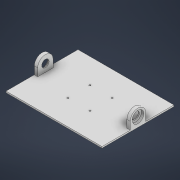
# Autodesk Inventor part: Testplatte_Differential
Saved by Autodesk Inventor 2021 (Build 250183000, 183)
## iProperties
Created: 2021-01-24
Part Number: Testplatte_Differential
Material: Generisch
Document SubType Name: Modeling
Designer: Ctroi
Density: 1 g/cm^3
Appearance: Vorgabe
Author: Ctroi
Autodesk Inventor part; units mm, degrees
ref_plane "YZ Plane" through (0, 0, 0) normal (1, 0, 0) x (0, 1, 0)
ref_plane "XZ Plane" through (0, 0, 0) normal (0, 1, 0) x (-1, 0, 0)
ref_plane "XY Plane" through (0, 0, 0) normal (0, 0, 1) x (1, 0, 0)
sketch "Skizze1" plane through (0, 0, 0) normal (0, 1, 0) x (-1, 0, 0)
  line L0 (100, -75) -> (-100, -75)
  line L1 (-100, -75) -> (-100, 75)
  line L2 (-100, 75) -> (100, 75)
  line L3 (100, 75) -> (100, -75)
  line L4 (0, -105) -> (0, 105) projected
  line L5 (-140, 0) -> (140, 0) projected
  point P0 (0, 0)
  dimension "d0" = 200
  dimension "d1" = 150
  constraints: 8 end point, 2 parallel, 1 horizontal, 1 perpendicular, 2 other
  measures "d0" distance of L1.end L2.end
  measures "d1" distance of L0.end L1.end
extrude "Extrusion1" add sketch "Skizze1" along normal blind 3
sketch "Skizze2" plane through (0, 3, 0) normal (0, 1, 0) x (1, 0, 0)
  line L0 (-93, 16) -> (-100, 16)
  line L1 (-100, 16) -> (-100, -16)
  line L2 (-100, -16) -> (-93, -16)
  line L3 (-93, -16) -> (-93, 16)
  line L4 (0, 105) -> (0, -105) projected
  line L5 (140, 0) -> (-140, 0) projected
  line L6 (-100, 75) -> (-100, -75) projected
  line L7 (93, 16) -> (100, 16)
  line L8 (100, 16) -> (100, -16)
  line L9 (100, -16) -> (93, -16)
  line L10 (93, -16) -> (93, 16)
  point P0 (0, 0)
  dimension "d4" = 7
  dimension "d5" = 32
  dimension "d6" = 0
  dimension "d58" = 32
  constraints: 16 end point, 4 symmetric about line, 2 parallel, 1 horizontal, 1 perpendicular, 1 other
  measures "d4" distance of L2.end L1.end
  measures "d5" distance of L1.end L0.end
  measures "d6" distance between parallel lines of L6 L1
  measures "d58" distance between parallel lines of L9 L7
extrude "Extrusion2" add sketch "Skizze2" along normal blind 32
sketch "Skizze3" plane through (-100, 0, -75) normal (-1, 0, 0) x (0, 0, 1)
  circle A0 centre (75, 19) radius 12.1
  line L0 (91, 3) -> (91, 35) projected
  line L1 (59, 35) -> (91, 35) projected
  point P0 (75, 0)
  dimension "d9" = 24.2
  dimension "d11" = 16
  dimension "d12" = 16
  constraints: 1 centre point
  measures "d9" diameter of A0
  measures "d11" distance from line of L0 A0.centre
  measures "d12" distance from line of L1 A0.centre
extrude "Extrusion4" cut sketch "Skizze3" against normal blind 5
sketch "Skizze4" plane through (100, 0, 75) normal (1, 0, 0) x (0, 0, -1)
  circle A0 centre (75, 19) radius 12.1
  line L0 (91, 3) -> (91, 35) projected
  line L1 (59, 35) -> (91, 35) projected
  point P0 (75, 0)
  dimension "d17" = 24.2
  dimension "d18" = 16
  dimension "d19" = 16
  constraints: 1 centre point
  measures "d17" diameter of A0
  measures "d18" distance from line of L0 A0.centre
  measures "d19" distance from line of L1 A0.centre
extrude "Extrusion5" cut sketch "Skizze4" against normal blind 5
sketch "Skizze5" plane through (95, 19, 0) normal (1, 0, 0) x (0, 0, -1)
  circle A0 centre (0, 0) radius 7.6
  line L0 (-16, 16) -> (16, 16) projected
  line L1 (-16, -16) -> (-16, 16) projected
  point P0 (0, -19)
  dimension "d22" = 15.2
  dimension "d23" = 16
  dimension "d24" = 16
  constraints: 1 centre point
  measures "d22" diameter of A0
  measures "d23" distance from line of L0 A0.centre
  measures "d24" distance from line of L1 A0.centre
sketch "Skizze6" plane through (-95, 19, 0) normal (-1, 0, 0) x (0, 0, 1)
  circle A0 centre (0, 0) radius 7.6
  line L0 (-16, 16) -> (16, 16) projected
  line L1 (16, -16) -> (16, 16) projected
  point P0 (0, -19)
  dimension "d25" = 15.2
  dimension "d26" = 16
  dimension "d27" = 16
  constraints: 1 centre point
  measures "d25" diameter of A0
  measures "d26" distance from line of L0 A0.centre
  measures "d27" distance from line of L1 A0.centre
extrude "Extrusion6" cut sketch "Skizze6" against normal up to surface (2 mm away)
extrude "Extrusion7" cut sketch "Skizze5" against normal up to surface (2 mm away)
sketch "Skizze11" plane through (0, 3, 0) normal (0, 1, 0) x (1, 0, 0)
  circle A0 centre (23, -23) radius 1.6
  circle A1 centre (23, 23) radius 1.6
  line L0 (140, 0) -> (-140, 0) projected
  line L1 (100, 16) -> (100, 75) projected
  line L2 (100, -75) -> (100, -16) projected
  line L3 (0, 105) -> (0, -105) projected
  circle A2 centre (-23, -23) radius 1.6
  circle A3 centre (-23, 23) radius 1.6
  circle A4 centre (23, 23) radius 1.6
  circle A5 centre (-23, 23) radius 1.6
  line L4 (100, 75) -> (-100, 75) projected
  point P0 (0, 0)
  dimension "d50" = 3.2
  dimension "d51" = 3.2
  dimension "d52" = 23
  dimension "d53" = 23
  dimension "d54" = 77
  dimension "d55" = 77
  dimension "d62" = 3.2
  dimension "d63" = 3.2
  dimension "d64" = 23
  dimension "d65" = 23
  dimension "d66" = 52
  dimension "d67" = 52
  constraints: 6 centre point, 2 symmetric about line, 2 other
  measures "d50" diameter of A0
  measures "d51" diameter of A1
  measures "d52" distance from line of L0 A0.centre
  measures "d53" distance from line of L0 A1.centre
  measures "d54" distance from line of L1 A1.centre
  measures "d55" distance from line of L2 A0.centre
  measures "d62" diameter of A4
  measures "d63" diameter of A5
  measures "d64" distance from line of L3 A4.centre
  measures "d65" distance from line of L3 A5.centre
  measures "d66" distance from line of L4 A5.centre
  measures "d67" distance from line of L4 A4.centre
extrude "Extrusion12" cut sketch "Skizze11" against normal up to surface (3 mm away) contours A0 | A1
fillet "Rundung1" radius 16 4 edges at (96.5, 35, -16) (96.5, 35, 16) (-96.5, 35, -16) (-96.5, 35, 16)
extrude "Extrusion13" cut sketch "Skizze11" against normal up to surface (3 mm away) contours A2 | A3
extrude "Extrusion14" cut sketch "Skizze11" against normal up to surface (3 mm away) contours A1 | A3
